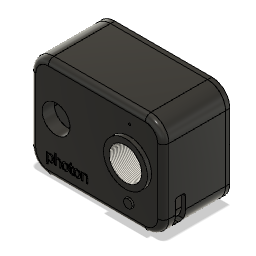
MDCEnclosure (Autodesk Fusion 360 design; units mm, degrees)
Autodesk Fusion 360 part; units mm, degrees
(part 1 of 2)
sketch "Board" plane through (0, 0, 0) normal (0, 0, 1) x (1, 0, 0)
  line L0 (4.75, 0) -> (39.105, 0)
  line L1 (43.855, 4.75) -> (43.855, 27.9)
  line L2 (39.105, 32.65) -> (4.75, 32.65)
  line L3 (0, 27.9) -> (0, 4.75)
  arc A0 (4.75, 32.65) -> (0, 27.9) centre (4.75, 27.9) ccw
  arc A1 (43.855, 27.9) -> (39.105, 32.65) centre (39.105, 27.9) ccw
  arc A2 (39.105, 0) -> (43.855, 4.75) centre (39.105, 4.75) ccw
  arc A3 (0, 4.75) -> (4.75, 0) centre (4.75, 4.75) ccw
  line L4 (-0.15, 27.9) -> (-0.15, 4.75)
  arc A4 (-0.15, 4.75) -> (4.75, -0.15) centre (4.75, 4.75) ccw
  line L5 (4.75, -0.15) -> (39.105, -0.15)
  arc A5 (39.105, -0.15) -> (44.005, 4.75) centre (39.105, 4.75) ccw
  line L6 (44.005, 4.75) -> (44.005, 27.9)
  arc A6 (44.005, 27.9) -> (39.105, 32.8) centre (39.105, 27.9) ccw
  line L7 (39.105, 32.8) -> (4.75, 32.8)
  arc A7 (4.75, 32.8) -> (-0.15, 27.9) centre (4.75, 27.9) ccw
  line L8 (-0.35, 27.9) -> (-0.35, 4.75)
  arc A8 (-0.35, 4.75) -> (4.75, -0.35) centre (4.75, 4.75) ccw
  line L9 (4.75, -0.35) -> (39.105, -0.35)
  arc A9 (39.105, -0.35) -> (44.205, 4.75) centre (39.105, 4.75) ccw
  line L10 (44.205, 4.75) -> (44.205, 27.9)
  arc A10 (44.205, 27.9) -> (39.105, 33) centre (39.105, 27.9) ccw
  line L11 (39.105, 33) -> (4.75, 33)
  arc A11 (4.75, 33) -> (-0.35, 27.9) centre (4.75, 27.9) ccw
  line L12 (-0.425, 27.9) -> (-0.425, 4.75)
  arc A12 (-0.425, 4.75) -> (4.75, -0.425) centre (4.75, 4.75) ccw
  line L13 (4.75, -0.425) -> (39.105, -0.425)
  arc A13 (39.105, -0.425) -> (44.28, 4.75) centre (39.105, 4.75) ccw
  line L14 (44.28, 4.75) -> (44.28, 27.9)
  arc A14 (44.28, 27.9) -> (39.105, 33.075) centre (39.105, 27.9) ccw
  line L15 (39.105, 33.075) -> (4.75, 33.075)
  arc A15 (4.75, 33.075) -> (-0.425, 27.9) centre (4.75, 27.9) ccw
  line L16 (21.9275, 32.65) -> (21.9275, 0)
  line L17 (21.9275, -0.425) -> (21.9275, 33.075)
  line L18 (21.9275, -0.35) -> (21.9275, 33)
  line L19 (43.855, 16.325) -> (0, 16.325)
  point P0 (21.9275, 16.325)
  dimension "d329" = 43.855
  dimension "d330" = 32.65
  dimension "d331" = 4.75
  dimension "d332" = 0.15
  dimension "d336" = 0.35
  dimension "d337" = 0.425
  dimension "d809" = 16.325
  constraint horizontal L0
  constraint vertical L1
  constraint horizontal L2
  constraint vertical L3
  constraint tangent L2 A0
  constraint tangent L3 A0
  constraint tangent L1 A1
  constraint tangent L2 A1
  constraint equal A0 A1
  constraint tangent L0 A2
  constraint tangent L1 A2
  constraint equal A0 A2
  constraint tangent L0 A3
  constraint tangent L3 A3
  constraint equal A0 A3
  constraint midpoint L2 L16.start
  constraint midpoint L0 L16.end
  constraint midpoint L16 P0
  constraint vertical L17
  constraint collinear L16 L17
  constraint vertical L18
  constraint collinear L16 L18
  constraint coincident L1 L19.start
  constraint coincident L3 L19.end
  constraint perpendicular L3 L19
  measures "d329" distance of L1 L3
  measures "d330" distance of L0 L2
  measures "d331" radius of A0
  measures "d809" distance of L0 L19
ref_plane "WorkPlane7" through (21.9275, 16.325, -3.46) normal (0, 0, 1) x (1, 0, 0)
sketch "MountPoints" plane through (0, 0, -3.46) normal (0, 0, 1) x (1, 0, 0)
  line L0 (-0.15, 27.9) -> (-0.15, 4.75)
  line L1 (4.75, -0.15) -> (39.105, -0.15)
  line L2 (3.44, 29.9) -> (0.44, 29.9)
  line L3 (0.44, 29.9) -> (0.44, 26.9)
  line L4 (0.44, 26.9) -> (3.44, 26.9)
  line L5 (3.44, 26.9) -> (3.44, 29.9)
  line L6 (3.44, 28.4) -> (0.44, 28.4)
  line L7 (0.44, 29.9) -> (-0.15, 29.9)
  line L8 (-0.15, 29.9) -> (-0.15, 26.9)
  line L9 (-0.15, 26.9) -> (0.44, 26.9)
  line L10 (0.44, 26.9) -> (0.44, 29.9)
  line L11 (3.182, 9.672) -> (0.182, 9.672)
  line L12 (0.182, 9.672) -> (0.182, 6.672)
  line L13 (0.182, 6.672) -> (3.182, 6.672)
  line L14 (3.182, 6.672) -> (3.182, 9.672)
  line L15 (3.182, 8.172) -> (0.182, 8.172)
  line L16 (0.182, 9.672) -> (-0.15, 9.672)
  line L17 (-0.15, 9.672) -> (-0.15, 6.672)
  line L18 (-0.15, 6.672) -> (0.182, 6.672)
  line L19 (0.182, 6.672) -> (0.182, 9.672)
  line L20 (44.4, 20.5) -> (39.4, 20.5)
  line L21 (39.4, 20.5) -> (39.4, 17.5)
  line L22 (39.4, 17.5) -> (44.4, 17.5)
  line L23 (44.4, 17.5) -> (44.4, 20.5)
  line L24 (44.4, 19) -> (39.4, 19)
  line L25 (44.005, 20.5) -> (44.4, 20.5)
  line L26 (44.4, 20.5) -> (44.4, 17.5)
  line L27 (44.4, 17.5) -> (44.005, 17.5)
  line L28 (44.005, 17.5) -> (44.005, 20.5)
  line L29 (44.005, 4.75) -> (44.005, 27.9)
  line L30 (0, 27.9) -> (0, 4.75)
  line L31 (4.75, 0) -> (39.105, 0)
  point P0 (1.94, 28.4)
  point P1 (1.682, 8.172)
  point P2 (41.9, 19)
  dimension "d662" = 3
  dimension "d663" = 3
  dimension "d664" = 3
  dimension "d665" = 3
  dimension "d666" = 3
  dimension "d667" = 5
  dimension "d668" = 1.682
  dimension "d669" = 8.172
  dimension "d670" = 1.94
  dimension "d671" = 28.4
  dimension "d672" = 19
  dimension "d673" = 41.9
  constraint horizontal L2
  constraint vertical L3
  constraint horizontal L4
  constraint vertical L5
  constraint midpoint L5 L6.start
  constraint midpoint L3 L6.end
  constraint midpoint P0 L6
  constraint horizontal L7
  constraint vertical L8
  constraint horizontal L9
  constraint vertical L10
  constraint collinear L0 L8
  constraint collinear L3 L10
  constraint collinear L2 L7
  constraint collinear L4 L9
  constraint horizontal L11
  constraint vertical L12
  constraint horizontal L13
  constraint vertical L14
  constraint midpoint L14 L15.start
  constraint midpoint L12 L15.end
  constraint midpoint P1 L15
  constraint horizontal L16
  constraint vertical L17
  constraint horizontal L18
  constraint vertical L19
  constraint collinear L0 L17
  constraint collinear L12 L19
  constraint collinear L11 L16
  constraint collinear L13 L18
  constraint horizontal L20
  constraint vertical L21
  constraint horizontal L22
  constraint vertical L23
  constraint midpoint L23 L24.start
  constraint midpoint L21 L24.end
  constraint midpoint P2 L24
  constraint horizontal L25
  constraint vertical L26
  constraint horizontal L27
  constraint vertical L28
  constraint collinear L28 L29
  constraint collinear L23 L26
  constraint collinear L20 L25
  constraint collinear L22 L27
  measures "d662" distance of L2 L4
  measures "d663" distance of L3 L5
  measures "d664" distance of L12 L14
  measures "d665" distance of L11 L13
  measures "d666" distance of L20 L22
  measures "d667" distance of L21 L23
  measures "d668" distance of P1 L30
  measures "d669" distance of P1 L31
  measures "d670" distance of P0 L30
  measures "d671" distance of P0 L31
  measures "d672" distance of P2 L31
  measures "d673" distance of P2 L30
sketch "BackplateMountPoints" plane through (0, 0, 0) normal (0, 0, 1) x (1, 0, 0)
  line L0 (44.005, 17.825) -> (42.505, 17.825)
  line L1 (42.505, 17.825) -> (42.505, 14.825)
  line L2 (42.505, 14.825) -> (44.005, 14.825)
  line L3 (44.005, 14.825) -> (44.005, 17.825)
  line L4 (44.005, 4.75) -> (44.005, 27.9)
  line L5 (4.75, 0) -> (39.105, 0)
  line L6 (1.35, 17.825) -> (-0.15, 17.825)
  line L7 (-0.15, 17.825) -> (-0.15, 14.825)
  line L8 (-0.15, 14.825) -> (1.35, 14.825)
  line L9 (1.35, 14.825) -> (1.35, 17.825)
  line L10 (-0.15, 27.9) -> (-0.15, 4.75)
  line L11 (44.005, 17.825) -> (44.005, 14.825)
  line L12 (-0.15, 17.825) -> (-0.15, 14.825)
  point P0 (42.505, 16.325)
  point P1 (1.35, 16.325)
  point P2 (44.005, 16.325)
  point P3 (-0.15, 16.325)
  dimension "d812" = 1.5
  dimension "d813" = 3
  dimension "d814" = 16.325
  dimension "d819" = 1.5
  dimension "d820" = 3
  dimension "d821" = 16.325
  dimension "d825" = 0
  dimension "d826" = 0
  constraint horizontal L0
  constraint vertical L1
  constraint horizontal L2
  constraint vertical L3
  constraint midpoint L1 P0
  constraint horizontal L6
  constraint vertical L7
  constraint horizontal L8
  constraint vertical L9
  constraint midpoint L9 P1
  constraint coincident L0 L3.end
  constraint coincident L2 L3.start
  constraint perpendicular L2 L11
  constraint midpoint L11 P2
  constraint collinear L3 L4
  constraint coincident L6 L7.start
  constraint coincident L8 L7.end
  constraint perpendicular L8 L12
  constraint midpoint L12 P3
  constraint collinear L7 L10
  measures "d812" distance of L1 L3
  measures "d813" distance of L0 L2
  measures "d814" distance of P0 L5
  measures "d819" distance of L7 L9
  measures "d820" distance of L6 L8
  measures "d821" distance of L5 P1
  measures "d825" distance of L3 L11
  measures "d826" distance of L7 L12
extrude "Front-Sidewalls" add sketch "Board" along normal blind 22.06 thin wall 1.5 on the left open curves L4 A4 L5 A5 L6 A6 L7 A7 makes body 1 in component "Front"
sketch "FrontHoles" plane through (0, 0, 0) normal (0, 0, 1) x (1, 0, 0)
  line L0 (0, 27.9) -> (0, 4.75)
  line L1 (4.75, 0) -> (39.105, 0)
  circle A0 centre (33.5424, 17.392) radius 7.5144
  circle A1 centre (33.5424, 17.392) radius 7.7644
  circle A2 centre (33.5424, 17.392) radius 6.8
  point P0 (7.5, 17.392)
  point P1 (33.5424, 17.392)
  point P2 (33.5424, 28.8)
  point P3 (33.5424, 4.75)
  dimension "d350" = 7.5
  dimension "d351" = 17.392
  dimension "d352" = 33.5424
  dimension "d353" = 17.392
  dimension "d554" = 15.0287
  dimension "d555" = 15.5287
  dimension "d575" = 13.6
  dimension "d647" = 33.5424
  dimension "d648" = 28.8
  dimension "d763" = 4.75
  dimension "d764" = 33.5424
  constraint coincident P1 A0.centre
  measures "d350" distance of P0 L0
  measures "d351" distance of P0 L1
  measures "d352" distance of P1 L0
  measures "d353" distance of P1 L1
  measures "d554" diameter of A0
  measures "d555" diameter of A1
  measures "d575" diameter of A2
  measures "d647" distance of L0 P2
  measures "d648" distance of L1 P2
  measures "d763" distance of L1 P3
  measures "d764" distance of L0 P3
sketch "Button" plane through (0, 0, 0) normal (0, 0, 1) x (1, 0, 0)
  circle A0 centre (33.5424, 4.75) radius 1.5
  circle A1 centre (33.5424, 4.75) radius 1.6
  circle A2 centre (33.5424, 4.75) radius 1.8
  point P0 (33.5424, 4.75)
  point P1 (33.5424, 4.75)
  dimension "d774" = 3
  dimension "d790" = 3.2
  dimension "d794" = 3.6
  constraint coincident P0 A0.centre
  constraint coincident P1 P0
  measures "d774" diameter of A0
  measures "d790" diameter of A1
  measures "d794" diameter of A2
extrude "Front-Frontplate" add sketch "Board" along normal blind 4.3 separate body contours L0 L3 A3 L16 L17 L18 L19 | L0 L2 L3 A0 A3 L4 A4 L5 L7 A7 L17 L18 | L0 L1 A2 L16 L17 L18 L19 | L0 L1 L2 A1 A2 L5 A5 L6 A6 L7 L17 L18 | L2 L3 A0 L16 L17 L18 L19 | L1 L2 A1 L16 L17 L18 L19 makes body 2 in component "Front"
hole "Front-MotionSensorHole" at (7.5, 17.392, 0) direction (0, 0, 1) diameter 9.9 depth 12 tip angle 118 bodies 2 in component "Front"
extrude "Front-LensProtrusionInside" [suppressed]
extrude "Extrude12" add sketch "FrontHoles" against normal blind 3.46 contours A0 | A2 bodies 2 in component "Front"
extrude "Front-BoardMountPoints" [suppressed]
extrude "Extrude16" add sketch "MountPoints" along normal blind 3.46 contours L0 L3 L7 L8 L9 L10 | L0 L16 L17 L18 L30 | L2 L3 L5 L6 L10 | L12 L16 L18 L19 L30 | L3 L4 L5 L6 L10 | L11 L12 L14 L15 L19 | L12 L13 L14 L15 L19 | L20 L23 L24 L25 L26 L28 L29 | L20 L21 L24 L28 L29 | L22 L23 L24 L26 L27 L28 L29 | L21 L22 L24 L28 L29 bodies 2 in component "Front"
extrude "Front-LensProtrusionBoardGap" cut sketch "FrontHoles" along normal blind 0.25 from surface at -3.46 contours A0 | A2 bodies 2 in component "Front"
extrude "Extrude24" [no effect]
extrude "Extrude18" cut sketch "FrontHoles" along normal blind 0.5 from surface at -3.21 contours A2 bodies 1 2 in component "Front"
extrude "Front-LensProtrusionOutside" [suppressed]
extrude "Extrude13" add sketch "FrontHoles" along normal blind 5.74 contours A0 | A1 | A2 bodies 2 in component "Front"
hole "Hole8" at (33.5424, 17.392, -2.71) direction (0, 0, 1) diameter 11.529 depth 20 tip angle 180 bodies 2 in component "Front"
thread "Thread2" "ISO Metric profile 12.0 M12x0.5 6H" major diameter 12.0961 minor diameter 11.5287 pitch 0.5 angle 60 resizes the face on face at (34.1164, 23.1279, 0.1067) from (33.5424, 17.392, -2.21) to (33.5424, 17.392, 5.74) on bodies 2 in component "Front"
hole "Hole10" at (1.94, 28.4, -3.46) at (1.682, 8.172, -3.46) at (41.9, 19, -3.46) direction (0, 0, 1) diameter 1.271 depth 5 tip angle 180 bodies 2 1 in component "Front"
thread "Thread4" "ISO Metric profile 1.6 M1.6x0.35 6H" major diameter 1.668 minor diameter 1.271 pitch 0.35 angle 60 resizes the face on face at (1.3283, 28.5721, -1.7933) on face at (1.7137, 8.8067, -1.7933) on face at (41.8683, 19.6347, -0.1267) on bodies 2 in component "Front"
hole "LEDHole" at (33.5424, 28.8, 0) direction (0, 0, 1) diameter 0.75 depth 4.3 tip angle 180 bodies 2 in component "Front"
hole "Hole12" at (33.5424, 4.75, 0) at (33.5424, 4.75, 0) direction (0, 0, 1) diameter 3.2 depth 4.3 tip angle 180 bodies 2 in component "Front"
move_body "MoveToFront" bodies 2 to x (1, 0, 0) y (0, 1, 0) z (0, 0, 1) at (0, 0, 17.76) in component "Front"
extrude "Extrude25" add sketch "BackplateMountPoints" along normal blind 22.06 separate body makes body 3 at (44.005, 15.825, 7.3533) makes body 4 at (-0.15, 16.825, 7.3533) in component "Front"
combine "Front-Combine" operation add target body 1 tool bodies 2 3 4 in component "Front"
hole "Hole13" at (44.005, 16.325, 0) at (-0.15, 16.325, 0) direction (0, 0, 1) diameter 1.271 depth 5 tip angle 180 bodies 1 in component "Front"
thread "Thread5" "ISO Metric profile 1.6 M1.6x0.35 6H" major diameter 1.668 minor diameter 1.271 pitch 0.35 angle 60 resizes the face on face at (43.9733, 16.9597, 3.3333) on face at (-0.7617, 16.4971, 1.6667) on bodies 1 in component "Front"
sketch "PhotonText" plane through (0, 0, 22.06) normal (0, 0, 1) x (1, 0, 0) in component "Front"
  spline S0 degree 3 poles (4.9102, 3.6944) (5.0407, 3.5604) (5.2188, 3.4933) (5.4446, 3.4933) knots 0 0 0 0 1 1 1 1
  spline S1 degree 3 poles (5.4446, 3.4933) (5.6704, 3.4933) (5.8344, 3.5692) (5.9367, 3.7209) knots 0 0 0 0 1 1 1 1
  spline S2 degree 3 poles (5.9367, 3.7209) (6.0391, 3.8726) (6.0902, 4.1001) (6.0902, 4.4035) knots 0 0 0 0 1 1 1 1
  line L0 (6.0902, 4.4035) -> (6.0902, 4.4141)
  spline S3 degree 3 poles (6.0902, 4.4141) (6.0902, 4.7139) (6.0408, 4.938) (5.942, 5.0861) knots 0 0 0 0 1 1 1 1
  spline S4 degree 3 poles (5.942, 5.0861) (5.8433, 5.2343) (5.6792, 5.3084) (5.4499, 5.3084) knots 0 0 0 0 1 1 1 1
  spline S5 degree 3 poles (5.4499, 5.3084) (5.2277, 5.3084) (5.0504, 5.2413) (4.9181, 5.1073) knots 0 0 0 0 1 1 1 1
  spline S6 degree 3 poles (4.9181, 5.1073) (4.7858, 4.9732) (4.7197, 4.7986) (4.7197, 4.5834) knots 0 0 0 0 1 1 1 1
  line L1 (4.7197, 4.5834) -> (4.7197, 4.2077)
  spline S7 degree 3 poles (4.7197, 4.2077) (4.7197, 4.0031) (4.7832, 3.832) (4.9102, 3.6944) knots 0 0 0 0 1 1 1 1
  spline S8 degree 3 poles (5.6034, 3.0065) (5.3847, 3.0065) (5.2012, 3.0488) (5.053, 3.1335) knots 0 0 0 0 1 1 1 1
  spline S9 degree 3 poles (5.053, 3.1335) (4.9049, 3.2182) (4.7973, 3.3258) (4.7303, 3.4563) knots 0 0 0 0 1 1 1 1
  line L2 (4.7303, 3.4563) -> (4.7197, 3.4563)
  line L3 (4.7197, 3.4563) -> (4.7197, 2.1704)
  line L4 (4.7197, 2.1704) -> (4.1323, 2.1704)
  line L5 (4.1323, 2.1704) -> (4.1323, 5.737)
  line L6 (4.1323, 5.737) -> (4.7038, 5.737)
  line L7 (4.7038, 5.737) -> (4.7197, 5.3401)
  line L8 (4.7197, 5.3401) -> (4.7303, 5.3401)
  spline S10 degree 3 poles (4.7303, 5.3401) (4.7867, 5.4601) (4.8925, 5.5668) (5.0477, 5.6603) knots 0 0 0 0 1 1 1 1
  spline S11 degree 3 poles (5.0477, 5.6603) (5.203, 5.7538) (5.3864, 5.8005) (5.5981, 5.8005) knots 0 0 0 0 1 1 1 1
  spline S12 degree 3 poles (5.5981, 5.8005) (5.9473, 5.8005) (6.2163, 5.6779) (6.4051, 5.4327) knots 0 0 0 0 1 1 1 1
  spline S13 degree 3 poles (6.4051, 5.4327) (6.5938, 5.1875) (6.6882, 4.848) (6.6882, 4.4141) knots 0 0 0 0 1 1 1 1
  line L9 (6.6882, 4.4141) -> (6.6882, 4.4035)
  spline S14 degree 3 poles (6.6882, 4.4035) (6.6882, 3.9555) (6.592, 3.6106) (6.3998, 3.369) knots 0 0 0 0 1 1 1 1
  spline S15 degree 3 poles (6.3998, 3.369) (6.2075, 3.1273) (5.942, 3.0065) (5.6034, 3.0065) knots 0 0 0 0 1 1 1 1
  line L10 (6.958, 3.07) -> (6.958, 6.7213)
  line L11 (6.958, 6.7213) -> (7.5454, 6.7213)
  line L12 (7.5454, 6.7213) -> (7.5454, 5.3401)
  line L13 (7.5454, 5.3401) -> (7.556, 5.3401)
  spline S16 degree 3 poles (7.556, 5.3401) (7.6195, 5.4707) (7.7227, 5.58) (7.8656, 5.6682) knots 0 0 0 0 1 1 1 1
  spline S17 degree 3 poles (7.8656, 5.6682) (8.0084, 5.7564) (8.1875, 5.8005) (8.4027, 5.8005) knots 0 0 0 0 1 1 1 1
  spline S18 degree 3 poles (8.4027, 5.8005) (8.699, 5.8005) (8.916, 5.7211) (9.0535, 5.5624) knots 0 0 0 0 1 1 1 1
  spline S19 degree 3 poles (9.0535, 5.5624) (9.1911, 5.4036) (9.2599, 5.1514) (9.2599, 4.8057) knots 0 0 0 0 1 1 1 1
  line L14 (9.2599, 4.8057) -> (9.2599, 3.07)
  line L15 (9.2599, 3.07) -> (8.6672, 3.07)
  line L16 (8.6672, 3.07) -> (8.6672, 4.8057)
  spline S20 degree 3 poles (8.6672, 4.8057) (8.6672, 4.9785) (8.6346, 5.102) (8.5694, 5.1761) knots 0 0 0 0 1 1 1 1
  spline S21 degree 3 poles (8.5694, 5.1761) (8.5041, 5.2502) (8.3938, 5.2872) (8.2386, 5.2872) knots 0 0 0 0 1 1 1 1
  spline S22 degree 3 poles (8.2386, 5.2872) (8.0093, 5.2872) (7.8365, 5.2219) (7.72, 5.0914) knots 0 0 0 0 1 1 1 1
  spline S23 degree 3 poles (7.72, 5.0914) (7.6036, 4.9609) (7.5454, 4.7968) (7.5454, 4.5993) knots 0 0 0 0 1 1 1 1
  line L17 (7.5454, 4.5993) -> (7.5454, 3.07)
  line L18 (7.5454, 3.07) -> (6.958, 3.07)
  spline S24 degree 3 poles (9.805, 5.4407) (10.0166, 5.6806) (10.3306, 5.8005) (10.7469, 5.8005) knots 0 0 0 0 1 1 1 1
  spline S25 degree 3 poles (10.7469, 5.8005) (11.1632, 5.8005) (11.4762, 5.6806) (11.6861, 5.4407) knots 0 0 0 0 1 1 1 1
  spline S26 degree 3 poles (11.6861, 5.4407) (11.896, 5.2008) (12.001, 4.8568) (12.001, 4.4088) knots 0 0 0 0 1 1 1 1
  line L19 (12.001, 4.4088) -> (12.001, 4.3982)
  spline S27 degree 3 poles (12.001, 4.3982) (12.001, 3.9502) (11.896, 3.6053) (11.6861, 3.3637) knots 0 0 0 0 1 1 1 1
  spline S28 degree 3 poles (11.6861, 3.3637) (11.4762, 3.122) (11.1632, 3.0012) (10.7469, 3.0012) knots 0 0 0 0 1 1 1 1
  spline S29 degree 3 poles (10.7469, 3.0012) (10.3306, 3.0012) (10.0175, 3.122) (9.8076, 3.3637) knots 0 0 0 0 1 1 1 1
  spline S30 degree 3 poles (9.8076, 3.3637) (9.5977, 3.6053) (9.4928, 3.9502) (9.4928, 4.3982) knots 0 0 0 0 1 1 1 1
  line L20 (9.4928, 4.3982) -> (9.4928, 4.4088)
  spline S31 degree 3 poles (9.4928, 4.4088) (9.4928, 4.8568) (9.5968, 5.2008) (9.805, 5.4407) knots 0 0 0 0 1 1 1 1
  spline S32 degree 3 poles (10.7469, 3.4933) (11.1878, 3.4933) (11.4083, 3.795) (11.4083, 4.3982) knots 0 0 0 0 1 1 1 1
  line L21 (11.4083, 4.3982) -> (11.4083, 4.4088)
  spline S33 degree 3 poles (11.4083, 4.4088) (11.4083, 5.0085) (11.1878, 5.3084) (10.7469, 5.3084) knots 0 0 0 0 1 1 1 1
  spline S34 degree 3 poles (10.7469, 5.3084) (10.3094, 5.3084) (10.0907, 5.0085) (10.0907, 4.4088) knots 0 0 0 0 1 1 1 1
  line L22 (10.0907, 4.4088) -> (10.0907, 4.3982)
  spline S35 degree 3 poles (10.0907, 4.3982) (10.0907, 3.795) (10.3094, 3.4933) (10.7469, 3.4933) knots 0 0 0 0 1 1 1 1
  line L23 (13.6308, 5.2555) -> (12.9588, 5.2555)
  line L24 (12.9588, 5.2555) -> (12.9588, 3.8108)
  spline S36 degree 3 poles (12.9588, 3.8108) (12.9588, 3.705) (12.9817, 3.6309) (13.0276, 3.5886) knots 0 0 0 0 1 1 1 1
  spline S37 degree 3 poles (13.0276, 3.5886) (13.0734, 3.5462) (13.1528, 3.5251) (13.2657, 3.5251) knots 0 0 0 0 1 1 1 1
  spline S38 degree 3 poles (13.2657, 3.5251) (13.3786, 3.5251) (13.5074, 3.541) (13.652, 3.5727) knots 0 0 0 0 1 1 1 1
  line L25 (13.652, 3.5727) -> (13.652, 3.1017)
  spline S39 degree 3 poles (13.652, 3.1017) (13.4827, 3.0488) (13.308, 3.0224) (13.1281, 3.0224) knots 0 0 0 0 1 1 1 1
  spline S40 degree 3 poles (13.1281, 3.0224) (12.8671, 3.0224) (12.6757, 3.0788) (12.554, 3.1917) knots 0 0 0 0 1 1 1 1
  spline S41 degree 3 poles (12.554, 3.1917) (12.4323, 3.3046) (12.3714, 3.5004) (12.3714, 3.7791) knots 0 0 0 0 1 1 1 1
  line L26 (12.3714, 3.7791) -> (12.3714, 5.2555)
  line L27 (12.3714, 5.2555) -> (12.0063, 5.2555)
  line L28 (12.0063, 5.2555) -> (12.0063, 5.737)
  line L29 (12.0063, 5.737) -> (12.3873, 5.737)
  line L30 (12.3873, 5.737) -> (12.4296, 6.499)
  line L31 (12.4296, 6.499) -> (12.9588, 6.499)
  line L32 (12.9588, 6.499) -> (12.9588, 5.737)
  line L33 (12.9588, 5.737) -> (13.6308, 5.737)
  line L34 (13.6308, 5.737) -> (13.6308, 5.2555)
  spline S42 degree 3 poles (14.0277, 5.4407) (14.2394, 5.6806) (14.5533, 5.8005) (14.9696, 5.8005) knots 0 0 0 0 1 1 1 1
  spline S43 degree 3 poles (14.9696, 5.8005) (15.3859, 5.8005) (15.699, 5.6806) (15.9089, 5.4407) knots 0 0 0 0 1 1 1 1
  spline S44 degree 3 poles (15.9089, 5.4407) (16.1188, 5.2008) (16.2238, 4.8568) (16.2238, 4.4088) knots 0 0 0 0 1 1 1 1
  line L35 (16.2238, 4.4088) -> (16.2238, 4.3982)
  spline S45 degree 3 poles (16.2238, 4.3982) (16.2238, 3.9502) (16.1188, 3.6053) (15.9089, 3.3637) knots 0 0 0 0 1 1 1 1
  spline S46 degree 3 poles (15.9089, 3.3637) (15.699, 3.122) (15.3859, 3.0012) (14.9696, 3.0012) knots 0 0 0 0 1 1 1 1
  spline S47 degree 3 poles (14.9696, 3.0012) (14.5533, 3.0012) (14.2403, 3.122) (14.0304, 3.3637) knots 0 0 0 0 1 1 1 1
  spline S48 degree 3 poles (14.0304, 3.3637) (13.8205, 3.6053) (13.7155, 3.9502) (13.7155, 4.3982) knots 0 0 0 0 1 1 1 1
  line L36 (13.7155, 4.3982) -> (13.7155, 4.4088)
  spline S49 degree 3 poles (13.7155, 4.4088) (13.7155, 4.8568) (13.8196, 5.2008) (14.0277, 5.4407) knots 0 0 0 0 1 1 1 1
  spline S50 degree 3 poles (14.9696, 3.4933) (15.4106, 3.4933) (15.6311, 3.795) (15.6311, 4.3982) knots 0 0 0 0 1 1 1 1
  line L37 (15.6311, 4.3982) -> (15.6311, 4.4088)
  spline S51 degree 3 poles (15.6311, 4.4088) (15.6311, 5.0085) (15.4106, 5.3084) (14.9696, 5.3084) knots 0 0 0 0 1 1 1 1
  spline S52 degree 3 poles (14.9696, 5.3084) (14.5322, 5.3084) (14.3135, 5.0085) (14.3135, 4.4088) knots 0 0 0 0 1 1 1 1
  line L38 (14.3135, 4.4088) -> (14.3135, 4.3982)
  spline S53 degree 3 poles (14.3135, 4.3982) (14.3135, 3.795) (14.5322, 3.4933) (14.9696, 3.4933) knots 0 0 0 0 1 1 1 1
  line L39 (16.4778, 3.07) -> (16.4778, 5.737)
  line L40 (16.4778, 5.737) -> (17.0493, 5.737)
  line L41 (17.0493, 5.737) -> (17.0651, 5.3348)
  line L42 (17.0651, 5.3348) -> (17.0757, 5.3348)
  spline S54 degree 3 poles (17.0757, 5.3348) (17.1427, 5.4654) (17.2468, 5.5756) (17.3879, 5.6656) knots 0 0 0 0 1 1 1 1
  spline S55 degree 3 poles (17.3879, 5.6656) (17.529, 5.7555) (17.7072, 5.8005) (17.9224, 5.8005) knots 0 0 0 0 1 1 1 1
  spline S56 degree 3 poles (17.9224, 5.8005) (18.2187, 5.8005) (18.4357, 5.7211) (18.5732, 5.5624) knots 0 0 0 0 1 1 1 1
  spline S57 degree 3 poles (18.5732, 5.5624) (18.7108, 5.4036) (18.7796, 5.1514) (18.7796, 4.8057) knots 0 0 0 0 1 1 1 1
  line L43 (18.7796, 4.8057) -> (18.7796, 3.07)
  line L44 (18.7796, 3.07) -> (18.187, 3.07)
  line L45 (18.187, 3.07) -> (18.187, 4.8057)
  spline S58 degree 3 poles (18.187, 4.8057) (18.187, 4.9785) (18.1543, 5.102) (18.0891, 5.1761) knots 0 0 0 0 1 1 1 1
  spline S59 degree 3 poles (18.0891, 5.1761) (18.0238, 5.2502) (17.9136, 5.2872) (17.7583, 5.2872) knots 0 0 0 0 1 1 1 1
  spline S60 degree 3 poles (17.7583, 5.2872) (17.529, 5.2872) (17.3562, 5.2219) (17.2397, 5.0914) knots 0 0 0 0 1 1 1 1
  spline S61 degree 3 poles (17.2397, 5.0914) (17.1233, 4.9609) (17.0651, 4.7951) (17.0651, 4.594) knots 0 0 0 0 1 1 1 1
  line L46 (17.0651, 4.594) -> (17.0651, 3.07)
  line L47 (17.0651, 3.07) -> (16.4778, 3.07)
  circle A0 centre (7.5, 17.392) radius 4.95
  circle A1 centre (33.5424, 17.392) radius 7.7643
  circle A2 centre (33.5424, 28.8) radius 0.375
  circle A3 centre (33.5424, 4.75) radius 1.6
  line L48 (-1.65, 27.9) -> (-1.65, 4.75)
  arc A4 (-1.65, 4.75) -> (4.75, -1.65) centre (4.75, 4.75) ccw
  line L49 (4.75, -1.65) -> (39.105, -1.65)
  arc A5 (39.105, -1.65) -> (45.505, 4.75) centre (39.105, 4.75) ccw
  line L50 (45.505, 4.75) -> (45.505, 27.9)
  arc A6 (45.505, 27.9) -> (39.105, 34.3) centre (39.105, 27.9) ccw
  line L51 (39.105, 34.3) -> (4.75, 34.3)
  arc A7 (4.75, 34.3) -> (-1.65, 27.9) centre (4.75, 27.9) ccw
extrude "Extrude26" cut sketch "PhotonText" against normal blind 0.25 contours S8 S9 L2 L3 L4 L5 L6 L7 L8 S10 S11 S12 S13 L9 S14 S15 | L10 L11 L12 L13 S16 S17 S18 S19 L14 L15 L16 S20 S21 S22 S23 L17 L18 | S24 S25 S26 L19 S27 S28 S29 S30 L20 S31 | L23 L24 S36 S37 S38 L25 S39 S40 S41 L26 L27 L28 L29 L30 L31 L32 L33 L34 | S42 S43 S44 L35 S45 S46 S47 S48 L36 S49 | L39 L40 L41 L42 S54 S55 S56 S57 L43 L44 L45 S58 S59 S60 S61 L46 L47 bodies 1 in component "Front"
fillet "Fillet20" radius 0.1 24 edges at (4.1323, 5.737, 21.935) (4.7038, 5.737, 21.935) (4.1323, 2.1704, 21.935) (4.7197, 2.1704, 21.935) (6.958, 6.7213, 21.935) (7.5454, 6.7213, 21.935) (6.958, 3.07, 21.935) (7.5454, 3.07, 21.935) (8.6672, 3.07, 21.935) (9.2599, 3.07, 21.935) (12.4296, 6.499, 21.935) (12.9588, 6.499, 21.935) (12.0063, 5.737, 21.935) (12.0063, 5.2555, 21.935) (13.6308, 5.737, 21.935) (13.6308, 5.2555, 21.935) (13.652, 3.5727, 21.935) (13.652, 3.1017, 21.935) (16.4778, 5.737, 21.935) (17.0493, 5.737, 21.935) (16.4778, 3.07, 21.935) (17.0651, 3.07, 21.935) (18.187, 3.07, 21.935) (18.7796, 3.07, 21.935) on bodies 1 in component "Front"
fillet "Fillet4" radius 1.5 8 edges at (3.44, 29.9, 16.03) (3.44, 26.9, 16.03) (3.182, 9.672, 16.03) (3.182, 6.672, 16.03) (42.505, 17.825, 7.15) (42.505, 14.825, 8.88) (1.35, 17.825, 8.88) (1.35, 14.825, 8.88) on bodies 1 in component "Front"
fillet "Fillet5" radius 1 9 edges at (-0.15, 26.9, 16.03) (0.2767, 29.9, 16.03) (44.005, 20.5, 16.03) (-0.15, 9.672, 16.03) (-0.15, 6.672, 16.03) (-0.15, 17.825, 8.88) (-0.15, 14.825, 8.88) (44.005, 17.825, 7.15) (44.005, 14.825, 8.88) on bodies 1 in component "Front"
fillet "Fillet16" radius 1 1 edges at (40.3839, 20.5, 16.155) on bodies 1 in component "Front"
fillet "Fillet17" radius 0.75 1 edges at (41.056, 17.5, 16.155) on bodies 1 in component "Front"
fillet "Fillet18" radius 0.75 1 edges at (43.0726, 17.5, 16.03) on bodies 1 in component "Front"
fillet "Fillet19" radius 1 2 edges at (40.3839, 20.5, 14.425) (41.056, 17.5, 14.425) on bodies 1 in component "Front"
fillet "FrontFillet" radius 2 8 edges at (-1.65, 16.325, 22.06) (0.2245, 0.2245, 22.06) (21.9275, -1.65, 22.06) (43.6305, 0.2245, 22.06) (45.505, 16.325, 22.06) (43.6305, 32.4255, 22.06) (21.9275, 34.3, 22.06) (0.2245, 32.4255, 22.06) on bodies 1 in component "Front"
extrude "Extrude1" add sketch "Button" along normal blind 7.66 separate body contours A0 makes body 5 in component "Button"
extrude "Extrude2" add sketch "Button" along normal blind 2.76 contours A0 | A1 | A2 bodies 5 in component "Button"
move_body "Align1" bodies 5 to x (1, 0, 0) y (0, 1, 0) z (0, 0, 1) at (0, 0, 14.4) in component "Button"
move_body "Move1" bodies 5 to x (1, 0, 0) y (0, 1, 0) z (0, 0, 1) at (0, 0, 0.6) in component "Button"
sketch "USBCPlugCutout" plane through (0, 0, 0) normal (1, 0, 0) x (0, 0, -1) in component "Front"
  line L0 (-22, 4.75) -> (-22, 27.9)
  line L1 (-22, 27.9) -> (-23.5, 27.9)
  line L2 (-23.5, 27.9) -> (-23.5, 4.75)
  line L3 (-23.5, 4.75) -> (-22, 4.75)
  line L4 (-18.715, 19.0109) -> (-17.155, 19.0109)
  line L5 (-16.155, 18.0109) -> (-16.155, 10.6709)
  line L6 (-17.155, 9.6709) -> (-18.715, 9.6709)
  line L7 (-19.715, 10.6709) -> (-19.715, 18.0109)
  arc A0 (-18.715, 19.0109) -> (-19.715, 18.0109) centre (-18.715, 18.0109) ccw
  arc A1 (-16.155, 18.0109) -> (-17.155, 19.0109) centre (-17.155, 18.0109) ccw
  arc A2 (-17.155, 9.6709) -> (-16.155, 10.6709) centre (-17.155, 10.6709) ccw
  arc A3 (-19.715, 10.6709) -> (-18.715, 9.6709) centre (-18.715, 10.6709) ccw
  dimension "d492" = 3.56
  dimension "d493" = 9.34
  dimension "d497" = 1
  dimension "d498" = 1
  dimension "d499" = 1
  constraint horizontal L4
  constraint vertical L5
  constraint vertical L7
  constraint tangent L4 A0
  constraint tangent L7 A0
  constraint tangent L4 A1
  constraint tangent L5 A1
  constraint tangent L5 A2
  constraint tangent L6 A2
  constraint tangent L6 A3
  constraint tangent L7 A3
  constraint equal A2 A3
  measures "d492" distance of L5 L7
  measures "d493" distance of L4 L6
  measures "d497" radius of A0
  measures "d498" radius of A1
  measures "d499" radius of A2
extrude "Extrude9" add sketch "USBCPlugCutout" along normal blind 10 separate body contours L4 L5 L6 L7 A0 A1 A2 A3 makes body 6 in component "Front"
ref_plane "WorkPlane5" through (42.1944, 19, 14.2) normal (0, 0, -1) x (-1, 0, 0) in component "Front"
ref_plane "WorkPlane6" through (42.005, 16.325, 11.03) normal (-1, 0, 0) x (0, -1, 0) in component "Front"
move_body "Align3" bodies 6 to x (1, 0, 0) y (0, 1, 0) z (0, 0, 1) at (42.005, 0, 0) in component "Front"
move_body "Align4" bodies 6 to x (1, 0, 0) y (0, 1, 0) z (0, 0, 1) at (0, 0, -1.955) in component "Front"
ref_plane "WorkPlane7" through (21.9275, 0, 0) normal (0, -1, 0) x (1, 0, 0) in component "Front"
ref_plane "WorkPlane9" through (21.9275, 5.2535, 0) normal (0, -1, 0) x (1, 0, 0) in component "Front"
move_body "Align5" bodies 6 to x (1, 0, 0) y (0, 1, 0) z (0, 0, 1) at (0, -9.0874, 0) in component "Front"
combine "Combine3" operation cut target body 1 tool bodies 6 in component "Front"
extrude "Extrude7" add sketch "Board" along normal blind 1.5 thin wall 1.5 on the left separate body open curves A4 L5 A5 L6 A6 L7 A7 L4 makes body 7 in component "Backplate"
extrude "Extrude8" add sketch "Board" along normal blind 1.5 contours L0 L3 A3 L16 L17 L18 L19 | L0 L2 L3 A0 A3 L4 A4 L5 L7 A7 L17 L18 | L0 L1 A2 L16 L17 L18 L19 | L0 L1 L2 A1 A2 L5 A5 L6 A6 L7 L17 L18 | L2 L3 A0 L16 L17 L18 L19 | L1 L2 A1 L16 L17 L18 L19 bodies 7 in component "Backplate"
move_body "Align11" bodies 7 to x (1, 0, 0) y (0, 1, 0) z (0, 0, 1) at (0, 0, -1.5) in component "Backplate"
sketch "Holes" plane through (0, 0, -1.5) normal (0, 0, -1) x (-1, 0, 0) in component "Backplate"
  arc A0 (-4.75, -1.65) -> (1.65, 4.75) centre (-4.75, 4.75) ccw
  line L0 (1.65, 4.75) -> (1.65, 27.9)
  arc A1 (1.65, 27.9) -> (-4.75, 34.3) centre (-4.75, 27.9) ccw
  line L1 (-4.75, 34.3) -> (-39.105, 34.3)
  arc A2 (-39.105, 34.3) -> (-45.505, 27.9) centre (-39.105, 27.9) ccw
  line L2 (-45.505, 27.9) -> (-45.505, 4.75)
  arc A3 (-45.505, 4.75) -> (-39.105, -1.65) centre (-39.105, 4.75) ccw
  line L3 (-39.105, -1.65) -> (-4.75, -1.65)
  point P0 (-44.005, 16.325)
  point P1 (-44.005, 16.325)
  point P2 (0.15, 16.325)
  point P3 (0.15, 16.325)
  constraint coincident P1 P0
  constraint coincident P3 P2
hole "Hole2" at (44.005, 16.325, -1.5) at (-0.15, 16.325, -1.5) direction (0, 0, 1) diameter 1.271 depth 1.5 tip angle 180 countersink diameter 3 countersink angle 90 bodies 7 in component "Backplate"
sketch "EngravingRect" plane through (0, 0, -1.5) normal (0, 0, -1) x (-1, 0, 0) in component "Backplate"
  arc A0 (-4.75, -1.65) -> (1.65, 4.75) centre (-4.75, 4.75) ccw
  line L0 (1.65, 4.75) -> (1.65, 16.325)
  circle A1 centre (0.15, 16.325) radius 1.5
  line L1 (1.65, 16.325) -> (1.65, 27.9)
  arc A2 (1.65, 27.9) -> (-4.75, 34.3) centre (-4.75, 27.9) ccw
  line L2 (-4.75, 34.3) -> (-39.105, 34.3)
  arc A3 (-39.105, 34.3) -> (-45.505, 27.9) centre (-39.105, 27.9) ccw
  line L3 (-45.505, 27.9) -> (-45.505, 16.325)
  circle A4 centre (-44.005, 16.325) radius 1.5
  line L4 (-45.505, 16.325) -> (-45.505, 4.75)
  arc A5 (-45.505, 4.75) -> (-39.105, -1.65) centre (-39.105, 4.75) ccw
  line L5 (-39.105, -1.65) -> (-4.75, -1.65)
  line L6 (-29.6775, 20.825) -> (-14.1775, 20.825)
  line L7 (-11.9275, 18.575) -> (-11.9275, 14.075)
  line L8 (-14.1775, 11.825) -> (-29.6775, 11.825)
  line L9 (-31.9275, 14.075) -> (-31.9275, 18.575)
  line L10 (-21.9275, -0.35) -> (-21.9275, 33)
  line L11 (-43.855, 16.325) -> (0, 16.325)
  arc A6 (-29.6775, 20.825) -> (-31.9275, 18.575) centre (-29.6775, 18.575) ccw
  arc A7 (-11.9275, 18.575) -> (-14.1775, 20.825) centre (-14.1775, 18.575) ccw
  arc A8 (-14.1775, 11.825) -> (-11.9275, 14.075) centre (-14.1775, 14.075) ccw
  arc A9 (-31.9275, 14.075) -> (-29.6775, 11.825) centre (-29.6775, 14.075) ccw
  dimension "d874" = 20
  dimension "d875" = 9
  dimension "d876" = 2.25
  constraint horizontal L6
  constraint vertical L7
  constraint horizontal L8
  constraint vertical L9
  constraint symmetric L7 L9 L10
  constraint symmetric L6 L8 L11
  constraint tangent L6 A6
  constraint tangent L9 A6
  constraint tangent L6 A7
  constraint tangent L7 A7
  constraint equal A6 A7
  constraint tangent L7 A8
  constraint tangent L8 A8
  constraint equal A6 A8
  constraint tangent L8 A9
  constraint tangent L9 A9
  constraint equal A6 A9
  measures "d874" distance of L7 L9
  measures "d875" distance of L6 L8
  measures "d876" radius of A6
extrude "Extrude9'" cut sketch "EngravingRect" against normal blind 0.25 contours L6 L7 L10 L11 A7 | L7 L8 L10 L11 A8 | L6 L9 L10 L11 A6 | L8 L9 L10 L11 A9 bodies 7 in component "Backplate"
sketch "ToasterText" plane through (0, 0, -1.25) normal (0, 0, -1) x (1, 0, 0) in component "Backplate"
  line L0 (27.7657, -16.7089) -> (28.4378, -16.7089)
  line L1 (28.4378, -16.7089) -> (28.4378, -15.2642)
  spline S0 degree 3 poles (28.4378, -15.2642) (28.4378, -15.1584) (28.4148, -15.0843) (28.369, -15.042) knots 0 0 0 0 1 1 1 1
  spline S1 degree 3 poles (28.369, -15.042) (28.3231, -14.9996) (28.2438, -14.9785) (28.1309, -14.9785) knots 0 0 0 0 1 1 1 1
  spline S2 degree 3 poles (28.1309, -14.9785) (28.018, -14.9785) (27.8892, -14.9944) (27.7446, -15.0261) knots 0 0 0 0 1 1 1 1
  line L2 (27.7446, -15.0261) -> (27.7446, -14.5551)
  spline S3 degree 3 poles (27.7446, -14.5551) (27.9139, -14.5022) (28.0885, -14.4758) (28.2684, -14.4758) knots 0 0 0 0 1 1 1 1
  spline S4 degree 3 poles (28.2684, -14.4758) (28.5295, -14.4758) (28.7209, -14.5322) (28.8426, -14.6451) knots 0 0 0 0 1 1 1 1
  spline S5 degree 3 poles (28.8426, -14.6451) (28.9643, -14.758) (29.0252, -14.9538) (29.0252, -15.2325) knots 0 0 0 0 1 1 1 1
  line L3 (29.0252, -15.2325) -> (29.0252, -16.7089)
  line L4 (29.0252, -16.7089) -> (29.3903, -16.7089)
  line L5 (29.3903, -16.7089) -> (29.3903, -17.1904)
  line L6 (29.3903, -17.1904) -> (29.0093, -17.1904)
  line L7 (29.0093, -17.1904) -> (28.9669, -17.9524)
  line L8 (28.9669, -17.9524) -> (28.4378, -17.9524)
  line L9 (28.4378, -17.9524) -> (28.4378, -17.1904)
  line L10 (28.4378, -17.1904) -> (27.7657, -17.1904)
  line L11 (27.7657, -17.1904) -> (27.7657, -16.7089)
  spline S6 degree 3 poles (27.3689, -16.8941) (27.1572, -17.134) (26.8432, -17.2539) (26.4269, -17.2539) knots 0 0 0 0 1 1 1 1
  spline S7 degree 3 poles (26.4269, -17.2539) (26.0107, -17.2539) (25.6976, -17.134) (25.4877, -16.8941) knots 0 0 0 0 1 1 1 1
  spline S8 degree 3 poles (25.4877, -16.8941) (25.2778, -16.6542) (25.1728, -16.3102) (25.1728, -15.8622) knots 0 0 0 0 1 1 1 1
  line L12 (25.1728, -15.8622) -> (25.1728, -15.8516)
  spline S9 degree 3 poles (25.1728, -15.8516) (25.1728, -15.4036) (25.2778, -15.0587) (25.4877, -14.8171) knots 0 0 0 0 1 1 1 1
  spline S10 degree 3 poles (25.4877, -14.8171) (25.6976, -14.5754) (26.0107, -14.4546) (26.4269, -14.4546) knots 0 0 0 0 1 1 1 1
  spline S11 degree 3 poles (26.4269, -14.4546) (26.8432, -14.4546) (27.1563, -14.5754) (27.3662, -14.8171) knots 0 0 0 0 1 1 1 1
  spline S12 degree 3 poles (27.3662, -14.8171) (27.5761, -15.0587) (27.6811, -15.4036) (27.6811, -15.8516) knots 0 0 0 0 1 1 1 1
  line L13 (27.6811, -15.8516) -> (27.6811, -15.8622)
  spline S13 degree 3 poles (27.6811, -15.8622) (27.6811, -16.3102) (27.577, -16.6542) (27.3689, -16.8941) knots 0 0 0 0 1 1 1 1
  spline S14 degree 3 poles (26.4269, -14.9467) (25.986, -14.9467) (25.7655, -15.2484) (25.7655, -15.8516) knots 0 0 0 0 1 1 1 1
  line L14 (25.7655, -15.8516) -> (25.7655, -15.8622)
  spline S15 degree 3 poles (25.7655, -15.8622) (25.7655, -16.4619) (25.986, -16.7618) (26.4269, -16.7618) knots 0 0 0 0 1 1 1 1
  spline S16 degree 3 poles (26.4269, -16.7618) (26.8644, -16.7618) (27.0831, -16.4619) (27.0831, -15.8622) knots 0 0 0 0 1 1 1 1
  line L15 (27.0831, -15.8622) -> (27.0831, -15.8516)
  spline S17 degree 3 poles (27.0831, -15.8516) (27.0831, -15.2484) (26.8644, -14.9467) (26.4269, -14.9467) knots 0 0 0 0 1 1 1 1
  line L16 (23.2996, -15.55) -> (23.2996, -15.7616)
  line L17 (23.2996, -15.7616) -> (23.7547, -15.7193)
  spline S18 degree 3 poles (23.7547, -15.7193) (24.0122, -15.6946) (24.1974, -15.6532) (24.3103, -15.595) knots 0 0 0 0 1 1 1 1
  spline S19 degree 3 poles (24.3103, -15.595) (24.4232, -15.5368) (24.4796, -15.43) (24.4796, -15.2748) knots 0 0 0 0 1 1 1 1
  line L18 (24.4796, -15.2748) -> (24.4796, -15.2642)
  spline S20 degree 3 poles (24.4796, -15.2642) (24.4796, -15.1513) (24.4435, -15.0649) (24.3711, -15.0049) knots 0 0 0 0 1 1 1 1
  spline S21 degree 3 poles (24.3711, -15.0049) (24.2988, -14.945) (24.1992, -14.915) (24.0722, -14.915) knots 0 0 0 0 1 1 1 1
  spline S22 degree 3 poles (24.0722, -14.915) (23.8393, -14.915) (23.6523, -14.9758) (23.5112, -15.0975) knots 0 0 0 0 1 1 1 1
  spline S23 degree 3 poles (23.5112, -15.0975) (23.3701, -15.2193) (23.2996, -15.3701) (23.2996, -15.55) knots 0 0 0 0 1 1 1 1
  line L19 (24.342, -16.3914) -> (24.9188, -16.3914)
  spline S24 degree 3 poles (24.9188, -16.3914) (24.9082, -16.663) (24.8086, -16.8738) (24.6198, -17.0237) knots 0 0 0 0 1 1 1 1
  spline S25 degree 3 poles (24.6198, -17.0237) (24.4311, -17.1736) (24.1515, -17.2486) (23.7811, -17.2486) knots 0 0 0 0 1 1 1 1
  spline S26 degree 3 poles (23.7811, -17.2486) (23.0756, -17.2486) (22.7228, -16.9523) (22.7228, -16.3596) knots 0 0 0 0 1 1 1 1
  line L20 (22.7228, -16.3596) -> (22.7228, -14.5234)
  line L21 (22.7228, -14.5234) -> (23.2572, -14.5234)
  line L22 (23.2572, -14.5234) -> (23.2731, -14.8991)
  line L23 (23.2731, -14.8991) -> (23.2837, -14.8991)
  spline S27 degree 3 poles (23.2837, -14.8991) (23.3578, -14.7686) (23.4733, -14.6627) (23.6303, -14.5816) knots 0 0 0 0 1 1 1 1
  spline S28 degree 3 poles (23.6303, -14.5816) (23.7873, -14.5005) (23.9681, -14.4599) (24.1727, -14.4599) knots 0 0 0 0 1 1 1 1
  spline S29 degree 3 poles (24.1727, -14.4599) (24.4408, -14.4599) (24.6551, -14.5234) (24.8156, -14.6504) knots 0 0 0 0 1 1 1 1
  spline S30 degree 3 poles (24.8156, -14.6504) (24.9761, -14.7774) (25.0564, -14.9714) (25.0564, -15.2325) knots 0 0 0 0 1 1 1 1
  line L24 (25.0564, -15.2325) -> (25.0564, -15.2431)
  spline S31 degree 3 poles (25.0564, -15.2431) (25.0564, -15.3771) (25.0344, -15.4935) (24.9903, -15.5923) knots 0 0 0 0 1 1 1 1
  spline S32 degree 3 poles (24.9903, -15.5923) (24.9462, -15.6911) (24.8888, -15.7705) (24.8183, -15.8304) knots 0 0 0 0 1 1 1 1
  spline S33 degree 3 poles (24.8183, -15.8304) (24.7477, -15.8904) (24.656, -15.9398) (24.5431, -15.9786) knots 0 0 0 0 1 1 1 1
  spline S34 degree 3 poles (24.5431, -15.9786) (24.4302, -16.0174) (24.3209, -16.0456) (24.215, -16.0633) knots 0 0 0 0 1 1 1 1
  spline S35 degree 3 poles (24.215, -16.0633) (24.1092, -16.0809) (23.9822, -16.0968) (23.834, -16.1109) knots 0 0 0 0 1 1 1 1
  line L25 (23.834, -16.1109) -> (23.3049, -16.1585)
  line L26 (23.3049, -16.1585) -> (23.3049, -16.3596)
  spline S36 degree 3 poles (23.3049, -16.3596) (23.3049, -16.5007) (23.3401, -16.6057) (23.4107, -16.6745) knots 0 0 0 0 1 1 1 1
  spline S37 degree 3 poles (23.4107, -16.6745) (23.4812, -16.7433) (23.6047, -16.7776) (23.7811, -16.7776) knots 0 0 0 0 1 1 1 1
  spline S38 degree 3 poles (23.7811, -16.7776) (24.1409, -16.7776) (24.3279, -16.6489) (24.342, -16.3914) knots 0 0 0 0 1 1 1 1
  spline S39 degree 3 poles (21.3364, -14.9256) (20.9836, -14.9256) (20.8072, -15.0402) (20.8072, -15.2695) knots 0 0 0 0 1 1 1 1
  line L27 (20.8072, -15.2695) -> (20.8072, -15.2801)
  spline S40 degree 3 poles (20.8072, -15.2801) (20.8072, -15.3789) (20.846, -15.4547) (20.9236, -15.5076) knots 0 0 0 0 1 1 1 1
  spline S41 degree 3 poles (20.9236, -15.5076) (21.0012, -15.5606) (21.1212, -15.5976) (21.2834, -15.6188) knots 0 0 0 0 1 1 1 1
  line L28 (21.2834, -15.6188) -> (21.5427, -15.6505)
  spline S42 degree 3 poles (21.5427, -15.6505) (21.8497, -15.6858) (22.0798, -15.7643) (22.2333, -15.886) knots 0 0 0 0 1 1 1 1
  spline S43 degree 3 poles (22.2333, -15.886) (22.3868, -16.0077) (22.4635, -16.1991) (22.4635, -16.4601) knots 0 0 0 0 1 1 1 1
  line L29 (22.4635, -16.4601) -> (22.4635, -16.4707)
  spline S44 degree 3 poles (22.4635, -16.4707) (22.4635, -16.7247) (22.3726, -16.9188) (22.191, -17.0528) knots 0 0 0 0 1 1 1 1
  spline S45 degree 3 poles (22.191, -17.0528) (22.0093, -17.1869) (21.7403, -17.2539) (21.384, -17.2539) knots 0 0 0 0 1 1 1 1
  spline S46 degree 3 poles (21.384, -17.2539) (20.689, -17.2539) (20.3239, -16.984) (20.2886, -16.4443) knots 0 0 0 0 1 1 1 1
  line L30 (20.2886, -16.4443) -> (20.8601, -16.4443)
  spline S47 degree 3 poles (20.8601, -16.4443) (20.8672, -16.5677) (20.913, -16.6559) (20.9977, -16.7089) knots 0 0 0 0 1 1 1 1
  spline S48 degree 3 poles (20.9977, -16.7089) (21.0824, -16.7618) (21.2111, -16.7882) (21.384, -16.7882) knots 0 0 0 0 1 1 1 1
  spline S49 degree 3 poles (21.384, -16.7882) (21.7227, -16.7882) (21.892, -16.6859) (21.892, -16.4813) knots 0 0 0 0 1 1 1 1
  line L31 (21.892, -16.4813) -> (21.892, -16.4707)
  spline S50 degree 3 poles (21.892, -16.4707) (21.892, -16.372) (21.8532, -16.297) (21.7756, -16.2458) knots 0 0 0 0 1 1 1 1
  spline S51 degree 3 poles (21.7756, -16.2458) (21.698, -16.1947) (21.571, -16.1585) (21.3946, -16.1374) knots 0 0 0 0 1 1 1 1
  line L32 (21.3946, -16.1374) -> (21.1512, -16.1056)
  spline S52 degree 3 poles (21.1512, -16.1056) (20.8337, -16.0597) (20.6017, -15.976) (20.4553, -15.8543) knots 0 0 0 0 1 1 1 1
  spline S53 degree 3 poles (20.4553, -15.8543) (20.3089, -15.7325) (20.2357, -15.5394) (20.2357, -15.2748) knots 0 0 0 0 1 1 1 1
  line L33 (20.2357, -15.2748) -> (20.2357, -15.2642)
  spline S54 degree 3 poles (20.2357, -15.2642) (20.2357, -14.7245) (20.6079, -14.4546) (21.3522, -14.4546) knots 0 0 0 0 1 1 1 1
  spline S55 degree 3 poles (21.3522, -14.4546) (22.1248, -14.4546) (22.5182, -14.7474) (22.5323, -15.333) knots 0 0 0 0 1 1 1 1
  line L34 (22.5323, -15.333) -> (21.9555, -15.333)
  spline S56 degree 3 poles (21.9555, -15.333) (21.9484, -15.199) (21.8893, -15.0975) (21.7782, -15.0288) knots 0 0 0 0 1 1 1 1
  spline S57 degree 3 poles (21.7782, -15.0288) (21.6671, -14.96) (21.5198, -14.9256) (21.3364, -14.9256) knots 0 0 0 0 1 1 1 1
  line L35 (18.5529, -16.7089) -> (19.225, -16.7089)
  line L36 (19.225, -16.7089) -> (19.225, -15.2642)
  spline S58 degree 3 poles (19.225, -15.2642) (19.225, -15.1584) (19.2021, -15.0843) (19.1562, -15.042) knots 0 0 0 0 1 1 1 1
  spline S59 degree 3 poles (19.1562, -15.042) (19.1103, -14.9996) (19.031, -14.9785) (18.9181, -14.9785) knots 0 0 0 0 1 1 1 1
  spline S60 degree 3 poles (18.9181, -14.9785) (18.8052, -14.9785) (18.6764, -14.9944) (18.5318, -15.0261) knots 0 0 0 0 1 1 1 1
  line L37 (18.5318, -15.0261) -> (18.5318, -14.5551)
  spline S61 degree 3 poles (18.5318, -14.5551) (18.7011, -14.5022) (18.8757, -14.4758) (19.0557, -14.4758) knots 0 0 0 0 1 1 1 1
  spline S62 degree 3 poles (19.0557, -14.4758) (19.3167, -14.4758) (19.5081, -14.5322) (19.6298, -14.6451) knots 0 0 0 0 1 1 1 1
  spline S63 degree 3 poles (19.6298, -14.6451) (19.7515, -14.758) (19.8124, -14.9538) (19.8124, -15.2325) knots 0 0 0 0 1 1 1 1
  line L38 (19.8124, -15.2325) -> (19.8124, -16.7089)
  line L39 (19.8124, -16.7089) -> (20.1775, -16.7089)
  line L40 (20.1775, -16.7089) -> (20.1775, -17.1904)
  line L41 (20.1775, -17.1904) -> (19.7965, -17.1904)
  line L42 (19.7965, -17.1904) -> (19.7542, -17.9524)
  line L43 (19.7542, -17.9524) -> (19.225, -17.9524)
  line L44 (19.225, -17.9524) -> (19.225, -17.1904)
  line L45 (19.225, -17.1904) -> (18.5529, -17.1904)
  line L46 (18.5529, -17.1904) -> (18.5529, -16.7089)
  spline S64 degree 3 poles (17.0395, -14.9361) (16.7855, -14.9361) (16.5033, -14.9908) (16.1929, -15.1002) knots 0 0 0 0 1 1 1 1
  line L47 (16.1929, -15.1002) -> (16.1929, -14.6239)
  spline S65 degree 3 poles (16.1929, -14.6239) (16.468, -14.5111) (16.7644, -14.4546) (17.0819, -14.4546) knots 0 0 0 0 1 1 1 1
  spline S66 degree 3 poles (17.0819, -14.4546) (17.5652, -14.4546) (17.9179, -14.571) (18.1402, -14.8039) knots 0 0 0 0 1 1 1 1
  spline S67 degree 3 poles (18.1402, -14.8039) (18.3624, -15.0367) (18.4736, -15.3859) (18.4736, -15.8516) knots 0 0 0 0 1 1 1 1
  line L48 (18.4736, -15.8516) -> (18.4736, -15.8622)
  spline S68 degree 3 poles (18.4736, -15.8622) (18.4736, -16.3067) (18.366, -16.6498) (18.1508, -16.8914) knots 0 0 0 0 1 1 1 1
  spline S69 degree 3 poles (18.1508, -16.8914) (17.9356, -17.1331) (17.6216, -17.2539) (17.2089, -17.2539) knots 0 0 0 0 1 1 1 1
  spline S70 degree 3 poles (17.2089, -17.2539) (16.4398, -17.2539) (16.0553, -16.8323) (16.0553, -15.9892) knots 0 0 0 0 1 1 1 1
  spline S71 degree 3 poles (16.0553, -15.9892) (16.0553, -15.8904) (16.0659, -15.774) (16.087, -15.6399) knots 0 0 0 0 1 1 1 1
  line L49 (16.087, -15.6399) -> (17.9021, -15.6399)
  spline S72 degree 3 poles (17.9021, -15.6399) (17.895, -15.3965) (17.8236, -15.2184) (17.6878, -15.1055) knots 0 0 0 0 1 1 1 1
  spline S73 degree 3 poles (17.6878, -15.1055) (17.5519, -14.9926) (17.3359, -14.9361) (17.0395, -14.9361) knots 0 0 0 0 1 1 1 1
  spline S74 degree 3 poles (16.7485, -16.6083) (16.8367, -16.7283) (16.9919, -16.7882) (17.2142, -16.7882) knots 0 0 0 0 1 1 1 1
  spline S75 degree 3 poles (17.2142, -16.7882) (17.4364, -16.7882) (17.6022, -16.7291) (17.7116, -16.611) knots 0 0 0 0 1 1 1 1
  spline S76 degree 3 poles (17.7116, -16.611) (17.8209, -16.4928) (17.8844, -16.3102) (17.9021, -16.0633) knots 0 0 0 0 1 1 1 1
  line L50 (17.9021, -16.0633) -> (16.6109, -16.0633)
  spline S77 degree 3 poles (16.6109, -16.0633) (16.6144, -16.3102) (16.6603, -16.4919) (16.7485, -16.6083) knots 0 0 0 0 1 1 1 1
  line L51 (15.8224, -14.5234) -> (15.8224, -17.1904)
  line L52 (15.8224, -17.1904) -> (15.2457, -17.1904)
  line L53 (15.2457, -17.1904) -> (15.2351, -16.6983)
  line L54 (15.2351, -16.6983) -> (15.2245, -16.6983)
  spline S78 degree 3 poles (15.2245, -16.6983) (15.1716, -16.8606) (15.0754, -16.9964) (14.9361, -17.1057) knots 0 0 0 0 1 1 1 1
  spline S79 degree 3 poles (14.9361, -17.1057) (14.7967, -17.2151) (14.6054, -17.261) (14.3619, -17.2433) knots 0 0 0 0 1 1 1 1
  line L55 (14.3619, -17.2433) -> (14.3619, -16.6612)
  spline S80 degree 3 poles (14.3619, -16.6612) (14.6724, -16.6612) (14.8955, -16.5969) (15.0313, -16.4681) knots 0 0 0 0 1 1 1 1
  spline S81 degree 3 poles (15.0313, -16.4681) (15.1672, -16.3393) (15.2351, -16.1268) (15.2351, -15.8304) knots 0 0 0 0 1 1 1 1
  line L56 (15.2351, -15.8304) -> (15.2351, -14.5234)
  line L57 (15.2351, -14.5234) -> (15.8224, -14.5234)
  arc A0 (29.6775, -20.825) -> (31.9275, -18.575) centre (29.6775, -18.575) ccw
  line L58 (31.9275, -18.575) -> (31.9275, -14.075)
  arc A1 (31.9275, -14.075) -> (29.6775, -11.825) centre (29.6775, -14.075) ccw
  line L59 (29.6775, -11.825) -> (14.1775, -11.825)
  arc A2 (14.1775, -11.825) -> (11.9275, -14.075) centre (14.1775, -14.075) ccw
  line L60 (11.9275, -14.075) -> (11.9275, -18.575)
  arc A3 (11.9275, -18.575) -> (14.1775, -20.825) centre (14.1775, -18.575) ccw
  line L61 (14.1775, -20.825) -> (29.6775, -20.825)
extrude "Extrude10" add sketch "ToasterText" along normal blind 0.25 contours L0 L1 S0 S1 S2 L2 S3 S4 S5 L3 L4 L5 L6 L7 L8 L9 L10 L11 | S6 S7 S8 L12 S9 S10 S11 S12 L13 S13 | L19 S24 S25 S26 L20 L21 L22 L23 S27 S28 S29 S30 L24 S31 S32 S33 S34 S35 L25 L26 S36 S37 S38 | S39 L27 S40 S41 L28 S42 S43 L29 S44 S45 S46 L30 S47 S48 S49 L31 S50 S51 L32 S52 S53 L33 S54 S55 L34 S56 S57 | L35 L36 S58 S59 S60 L37 S61 S62 S63 L38 L39 L40 L41 L42 L43 L44 L45 L46 | S64 L47 S65 S66 S67 L48 S68 S69 S70 S71 L49 S72 S73 | L51 L52 L53 L54 S78 S79 L55 S80 S81 L56 L57 bodies 7 in component "Backplate"
fillet "Fillet6" radius 0.1 13 edges at (29.0093, 17.1904, -1.375) (28.4378, 17.1904, -1.375) (29.0252, 16.7089, -1.375) (28.4378, 16.7089, -1.375) (23.2996, 15.7616, -1.375) (23.2731, 14.8991, -1.375) (19.7965, 17.1904, -1.375) (19.225, 17.1904, -1.375) (19.8124, 16.7089, -1.375) (19.225, 16.7089, -1.375) (17.9021, 16.0633, -1.375) (16.6109, 16.0633, -1.375) (15.2351, 16.6983, -1.375) on bodies 7 in component "Backplate"